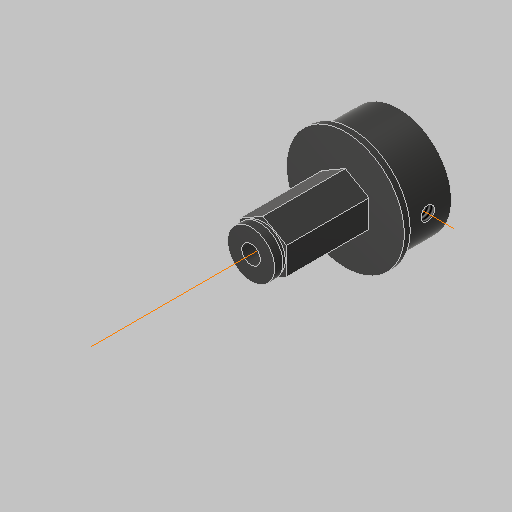
# Autodesk Inventor part: WCP-0102
Saved by Autodesk Inventor 2023.5 (Build 275446000, 446)
## iProperties
Created: 2019-02-02
Part Number: WCP-0102
Material: Aluminum 6061
Document SubType Name: Modeling
Designer: pctech
Density: 2.7 g/cm^3
Appearance: Smooth - Black
Mass: 32.1877 g
Surface Area: 48.0979 cm^2
Volume: 11.9214 cm^3
Author: pctech
Autodesk Inventor part; units mm, degrees
ref_plane "YZ Plane" through (0, 0, 0) normal (1, 0, 0) x (0, 1, 0)
ref_plane "XZ Plane" through (0, 0, 0) normal (0, 1, 0) x (-1, 0, 0)
sketch "Sketch1" plane through (0, 0, 0) normal (0, 0, 1) x (1, 0, 0)
  line L0 (0, 7.3323) -> (6.35, 3.6662)
  line L1 (6.35, 3.6662) -> (6.35, -3.6662)
  line L2 (6.35, -3.6662) -> (0, -7.3323)
  line L3 (0, -7.3323) -> (-6.35, -3.6662)
  line L4 (-6.35, -3.6662) -> (-6.35, 3.6662)
  line L5 (-6.35, 3.6662) -> (0, 7.3323)
  point P0 (0, 0)
  point P1 (0, 0)
  dimension "d0" = 12.7
  constraints: 12 end point, 1 coincident, 1 vertical alignment, 13 other
  measures "d0" distance between parallel lines of L1 L4
extrude "Extrusion1" add sketch "Sketch1" along normal blind 25.4
sketch "Sketch2" plane through (0, 0, 0) normal (0, 0, -1) x (-1, 0, 0)
  circle A0 centre (0, 0) radius 15.875
  dimension "d3" = 31.75
  constraints: 1 centre point, 1 coincident
  measures "d3" diameter of A0
extrude "Extrusion2" add sketch "Sketch2" along normal blind 1.5875
sketch "Sketch3" plane through (0, 0, -1.5875) normal (0, 0, -1) x (-1, 0, 0)
  circle A0 centre (0, 0) radius 14.2875
  dimension "d6" = 28.575
  constraints: 1 centre point, 1 coincident
  measures "d6" diameter of A0
extrude "Extrusion3" add sketch "Sketch3" along normal blind 12.7
sketch "Sketch4" plane through (0, 0, -14.2875) normal (0, 0, -1) x (-1, 0, 0)
  circle A0 centre (0, 0) radius 14.2875 construction
  constraints: 1 coincident
hole "Hole1" at (0, 0, -14.2875) direction (0, 0, 1) diameter 4.9784 end through all thread size "1/4-20 UNC" class "2B" standard "ANSI Unified Screw Threads"
ref_plane "Work Plane1" through (14.2875, 0, -1.5875) normal (1, 0, 0) x (0, 1, 0)
sketch "Sketch5" plane through (14.2875, 0, -1.5875) normal (1, 0, 0) x (0, 1, 0)
  line L0 (-14.2875, -12.7) -> (14.2875, -12.7) construction
  line L1 (14.2875, 0) -> (-14.2875, 0) construction
  line L2 (14.2875, 0) -> (14.2875, -12.7) construction
  line L3 (14.2875, 0) -> (14.2875, -12.7) construction
  point P0 (0, 1.5875)
  point P1 (0, -6.35)
  point P2 (14.2875, -6.35)
  constraints: 2 end point, 1 collinear, 1 horizontal alignment, 1 midpoint, 1 vertical alignment
hole "Hole2" at (14.2875, 0, -7.9375) direction (-1, 0, 0) diameter 3.683 depth 9.525 thread size "10-24 UNC" class "2B" standard "ANSI Unified Screw Threads"
mirror "Mirror1" about plane through (0, 0, 0) normal (1, 0, 0) of "Hole2"
sketch "Sketch6" plane through (0, 0, 25.4) normal (0, 0, 1) x (1, 0, 0)
  circle A0 centre (0, 0) radius 6.35
  circle A1 centre (0, 0) radius 15.875 construction
  line L0 (6.35, 3.6662) -> (6.35, -3.6662) construction
  line L1 (6.35, -3.6662) -> (0, -7.3323) construction
  line L2 (0, -7.3323) -> (-6.35, -3.6662) construction
  line L3 (-6.35, -3.6662) -> (-6.35, 3.6662) construction
  line L4 (-6.35, 3.6662) -> (0, 7.3323) construction
  line L5 (0, 7.3323) -> (6.35, 3.6662) construction
  line L6 (0, 7.3323) -> (6.35, 3.6662)
  line L7 (6.35, 3.6662) -> (6.35, -3.6662)
  line L8 (6.35, -3.6662) -> (0, -7.3323)
  line L9 (0, -7.3323) -> (-6.35, -3.6662)
  line L10 (-6.35, -3.6662) -> (-6.35, 3.6662)
  line L11 (-6.35, 3.6662) -> (0, 7.3323)
  constraints: 12 end point, 2 coincident, 1 centre point, 1 tangent, 13 other
extrude "Extrusion4" cut sketch "Sketch6" against normal blind 3.175 contours L7 L8 A0 | A0 L6 L7 | A0 L11 L6 | L8 L9 A0 | A0 L10 L11 | L9 L10 A0
sketch "Sketch7" plane through (0, 0, 0) normal (1, 0, 0) x (0, 1, 0)
  line L0 (14.2875, -1.5875) -> (14.2875, -14.2875) construction
  line L1 (14.2875, -14.2875) -> (2.4892, -14.2875) construction
  line L2 (2.4892, -14.2875) -> (2.4892, 25.4) construction
  line L3 (2.4892, 25.4) -> (6.35, 25.4) construction
  line L4 (6.35, 25.4) -> (6.35, 22.225) construction
  line L5 (6.35, 22.225) -> (7.3323, 22.225) construction
  line L6 (7.3323, 22.225) -> (7.3323, 0) construction
  line L7 (7.3323, 0) -> (15.875, 0) construction
  line L8 (15.875, 0) -> (15.875, -1.5875) construction
  line L9 (15.875, -1.5875) -> (14.2875, -1.5875) construction
  line L10 (-15.875, 0) -> (-7.3323, 0) construction
  line L11 (-7.3323, 0) -> (-7.3323, 22.225) construction
  line L12 (-7.3323, 22.225) -> (-6.35, 22.225) construction
  line L13 (-6.35, 22.225) -> (-6.35, 25.4) construction
  line L14 (-6.35, 25.4) -> (-2.4892, 25.4) construction
  line L15 (-2.4892, 25.4) -> (-2.4892, -14.2875) construction
  line L16 (-2.4892, -14.2875) -> (-14.2875, -14.2875) construction
  line L17 (-14.2875, -14.2875) -> (-14.2875, -1.5875) construction
  line L18 (-14.2875, -1.5875) -> (-15.875, -1.5875) construction
  line L19 (-15.875, -1.5875) -> (-15.875, 0) construction
  line L20 (6.35, 22.225) -> (6.0325, 22.225)
  line L21 (6.0325, 22.225) -> (6.0325, 23.1775)
  line L22 (6.0325, 23.1775) -> (6.35, 23.1775)
  line L23 (6.35, 23.1775) -> (6.35, 22.225)
  line L24 (0, -22.225) -> (0, 33.3375) projected
  point P0 (0, 0)
  dimension "d25" = 0.3175
  dimension "d26" = 0.9525
  constraints: 8 end point, 2 parallel, 1 horizontal, 1 perpendicular
  measures "d25" distance between parallel lines of L4 L21
  measures "d26" distance between parallel lines of L20 L22
revolve "Revolution1" cut sketch "Sketch7" angle 360 about axis through (0, 0, -10) along (0, 0, 1)
sketch "Sketch8" plane through (0, 0, 25.4) normal (0, 0, 1) x (1, 0, 0)
  circle A0 centre (0, 0) radius 6.35 projected
  circle A1 centre (0, 0) radius 2.4892 projected
  circle A2 centre (0, 0) radius 15.875 projected
  line L0 (6.35, 3.6662) -> (6.35, -3.6662) projected
  line L1 (6.35, -3.6662) -> (0, -7.3323) projected
  line L2 (0, -7.3323) -> (-6.35, -3.6662) projected
  line L3 (-6.35, -3.6662) -> (-6.35, 3.6662) projected
  line L4 (-6.35, 3.6662) -> (0, 7.3323) projected
  line L5 (0, 7.3323) -> (6.35, 3.6662) projected
extrude "Extrusion5" [suppressed]
body "Solid1"
